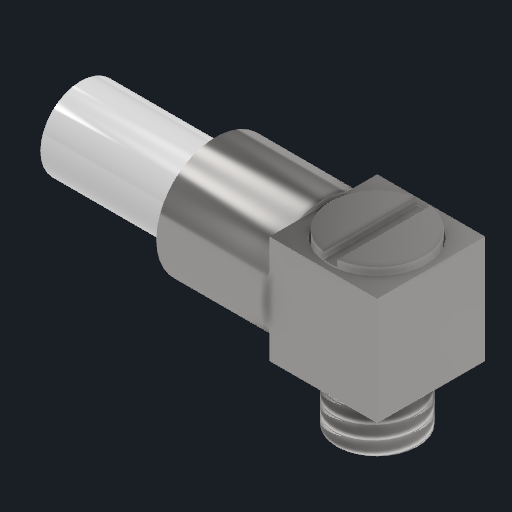
# Autodesk Inventor part: 6mm hose fitting
Saved by Autodesk Inventor 2024.3 (Build 283343000, 343)
## iProperties
Created: 2024-09-28
Part Number: 6mm hose fitting
Material: Generic
Document SubType Name: Modeling
Designer: MFil
Density: 4.67513 g/cm^3
Appearance: Default
Mass: 6 g
Surface Area: 10.4185 cm^2
Volume: 1.28339 cm^3
Author: MFil
Autodesk Inventor part; units mm, degrees
ref_plane "YZ Plane" through (0, 0, 0) normal (1, 0, 0) x (0, 1, 0)
ref_plane "XZ Plane" through (0, 0, 0) normal (0, 1, 0) x (-1, 0, 0)
ref_plane "XY Plane" through (0, 0, 0) normal (0, 0, 1) x (1, 0, 0)
sketch "Sketch1" plane through (0, 0, 0) normal (0, 1, 0) x (-1, 0, 0)
  line L0 (0, 0) -> (8, 0)
  line L1 (8, 0) -> (8, -4.4)
  line L2 (8, -4.4) -> (0, -4.4)
  line L3 (0, -4.4) -> (0, 0)
  line L4 (0, 0) -> (-8, 0)
  line L5 (-8, 0) -> (-8, -4)
  line L6 (-8, -4) -> (0, -4)
  line L7 (0, -4) -> (0, 0)
  line L8 (-8, 0) -> (0, 0)
  line L9 (0, 0) -> (0, 4)
  line L10 (0, 4) -> (-8, 4)
  line L11 (-8, 4) -> (-8, 0)
  circle A0 centre (-4, 0) radius 3
  line L12 (8, -2) -> (18, -2)
  line L13 (18, -2) -> (18, -3)
  line L14 (18, -3) -> (8, -3)
  line L15 (8, -3) -> (8, -2)
  circle A1 centre (-4, 0) radius 3.5
  line L16 (-3.5, 3.6063) -> (-4.5, 3.6063)
  line L17 (-4.5, 3.6063) -> (-4.5, -3.6063)
  line L18 (-4.5, -3.6063) -> (-3.5, -3.6063)
  line L19 (-3.5, -3.6063) -> (-3.5, 3.6063)
  line L20 (-3.5, 3.6063) -> (-4.5, -3.6063) construction
  line L21 (-4.5, 3.6063) -> (-3.5, -3.6063) construction
  point P0 (-4.5, 3.4641)
  point P1 (-4.5, -3.4641)
  point P2 (-3.5, -3.4641)
  point P3 (-3.5, 3.4641)
  dimension "d0" = 8
  dimension "d1" = 4.4
  dimension "d2" = 8
  dimension "d3" = 4
  dimension "d4" = 4
  dimension "d5" = 6
  dimension "d6" = 10
  dimension "d7" = 1
  dimension "d8" = 2
  dimension "d9" = 7
  dimension "d10" = 1
  constraints: 44 end point, 10 parallel, 5 horizontal, 5 perpendicular, 3 midpoint, 2 centre point, 2 point on line, 1 coincident
  measures "d0" distance of L1.end L2.end
  measures "d1" distance of L0.end L1.end
  measures "d2" distance of L6.end L5.end
  measures "d3" distance of L5.end L4.end
  measures "d4" distance of L9.end L8.end
  measures "d5" diameter of A0
  measures "d6" distance of L13.end L14.end
  measures "d7" distance of L12.end L13.end
  measures "d8" distance between parallel lines of L0 L12
  measures "d9" diameter of A1
  measures "d10" distance of L18.end L17.end
revolve "Revolution1" add sketch "Sketch1" angle 360 about axis through (0, 0, 0) along (-1, 0, 0) contours L0 L1 L2 L3
revolve "Revolution2" add sketch "Sketch1" angle 360 about axis through (0, 0, 0) along (-1, 0, 0) contours L12 L13 L14 L1
extrude "Extrusion1" add sketch "Sketch1" along normal mid plane 8 contours L3 L6 L5 L4 A1 L17 L18 L19 | L4 A1 L19 L16 L17 L11 L10 L9 | A1 L19 A0 L4 | L4 A0 L19 A1 | A0 L19 L4 | L4 L19 A0 | L19 A0 L17 A1 | A1 L17 L16 L19 | L19 L18 L17 A1 | A1 L17 A0 L19 | L19 A0 L17 L4 | L4 L17 A0 L19 | L17 A0 L4 A1 | A1 L4 A0 L17 | L17 A0 L4 | L4 A0 L17
extrude "Extrusion2" add sketch "Sketch1" against normal blind 8 contours A0 L19 L4 | L4 L19 A0 | L19 A0 L17 L4 | L4 L17 A0 L19 | L17 A0 L4 | L4 A0 L17
extrude "Extrusion3" add sketch "Sketch1" along normal blind 4.5 contours A1 L19 A0 L4 | L4 A0 L19 A1 | A0 L19 L4 | L4 L19 A0 | L17 A0 L4 A1 | A1 L4 A0 L17 | L17 A0 L4 | L4 A0 L17
sketch "Sketch2" plane through (0, 4, 0) normal (0, 1, 0) x (1, 0, 0)
  arc A0 (3.5, 3.4641) -> (3.5, -3.4641) centre (4, 0) ccw projected
  line L0 (3.5, -3.4641) -> (3.5, 3.4641) projected
  arc A1 (4.5, -3.4641) -> (4.5, 3.4641) centre (4, 0) ccw projected
  line L1 (4.5, 3.4641) -> (4.5, -3.4641) projected
  line L2 (4.5, -3.4641) -> (4.5, 3.4641) projected
  arc A2 (4.5, -3.4641) -> (4.5, 3.4641) centre (4, 0) ccw projected
  line L3 (3.5, 3.4641) -> (3.5, -3.4641) projected
  arc A3 (3.5, 3.4641) -> (3.5, -3.4641) centre (4, 0) ccw projected
  line L4 (0, -4) -> (8, -4) projected
  line L5 (8, -4) -> (8, 4) projected
  line L6 (8, 4) -> (0, 4) projected
  line L7 (0, 4) -> (0, 1.833) projected
  line L8 (0, -1.833) -> (0, 1.833) projected
  line L9 (0, -1.833) -> (0, -4) projected
  circle A4 centre (4, 0) radius 3.6
  circle A5 centre (4, 0) radius 3.5
  point P0 (0, 0)
  point P1 (3.5, -3.4641)
  dimension "d19" = 7.2
  constraints: 2 coincident, 1 centre point, 3 other
  measures "d19" diameter of A4
extrude "Extrusion4" cut sketch "Sketch2" against normal blind 0.5 contours A4
thread "Thread1" size "M6x1" class "6g" standard "ISO Metric profile" length 3.5 offset 0.5
body "Solid1"
